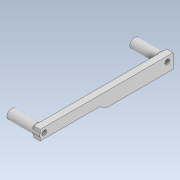
# Autodesk Inventor part: PCB_support
Saved by Autodesk Inventor 2020 (Build 240168000, 168)
## iProperties
Created: 2021-04-10
Part Number: PCB_support
Material: Generic
Document SubType Name: Modeling
Designer: DELL
Density: 1 g/cm^3
Appearance: Default
Author: DELL
Autodesk Inventor part; units mm, degrees
ref_plane "YZ Plane" through (0, 0, 0) normal (1, 0, 0) x (0, 1, 0)
ref_plane "XZ Plane" through (0, 0, 0) normal (0, 1, 0) x (-1, 0, 0)
ref_plane "XY Plane" through (0, 0, 0) normal (0, 0, 1) x (1, 0, 0)
sketch "Sketch1" plane through (0, 0, 0) normal (1, 0, 0) x (0, 1, 0)
  line L0 (5, -46.5) -> (-5, -46.5)
  line L1 (-5, -46.5) -> (-5, 46.5)
  line L2 (-5, 46.5) -> (5, 46.5)
  line L3 (5, 46.5) -> (5, -46.5)
  line L4 (5, -46.5) -> (-5, 46.5) construction
  line L5 (-5, -46.5) -> (5, 46.5) construction
  circle A0 centre (1.5, 43.5) radius 1.25
  circle A1 centre (1.5, -42.5) radius 1.25
  line L6 (-2, 46.5) -> (-2, 5)
  line L7 (-2, 5) -> (-5, 0)
  point P0 (0, 0)
  dimension "d0" = 2.5
  dimension "d2" = 86
  dimension "d3" = 93
  dimension "d4" = 3.5
  dimension "d5" = 6.5
  dimension "d6" = 4
  dimension "d20" = 3.5
  dimension "d21" = 5
  constraints: 16 end point, 3 midpoint, 2 centre point, 2 parallel, 2 perpendicular, 1 equal radius, 1 horizontal, 1 point on line, 1 vertical alignment
  measures "d0" diameter of A0
  measures "d2" distance of A1.centre A0.centre
  measures "d3" distance of L2.end L0.start
  measures "d4" distance from line of A0.centre L3
  measures "d5" distance from line of A0.centre L1
  measures "d6" distance from line of L0 A1.centre
  measures "d20" distance from line of A0.centre L6
  measures "d21" vertical distance of L6.end L7.end
extrude "Extrusion1" add sketch "Sketch1" along normal blind 4.5 contours L0 L1 L7 L6 L2 L3
sketch "Sketch2" plane through (4.5, 0, 0) normal (1, 0, 0) x (0, 0, -1)
  circle A0 centre (-43.5, 1.5) radius 1.25 projected
  circle A1 centre (-43.5, 1.5) radius 3.25
  circle A2 centre (42.5, 1.5) radius 1.25 projected
  circle A3 centre (42.5, 1.5) radius 3.25
  point P0 (0, 0)
  dimension "d9" = 6.5
  constraints: 2 centre point, 2 coincident, 1 equal radius
  measures "d9" diameter of A1
extrude "Extrusion2" add sketch "Sketch2" against normal blind 23
fillet "Fillet1" radius 1 3 edges at (0, -1.6869, 42.8626) (0, 4.6869, 42.8626) (0, 1.5, -39.25)
chamfer "Chamfer1" distance 0.5 angle 45 6 edges at (4.5, 0.6161, 44.3839) (4.5, 2.3839, 42.6161) (4.5, 2.3839, -43.3839) (4.5, 0.6161, -41.6161) (-18.5, 1.5, -41.25) (-18.5, 1.5, 44.75)
body "Solid1"
